Autodesk Fusion 360 part; units mm, degrees
(part 2 of 6)
  line L465 (-177.5, -38.5) -> (-158.5, -57.5) construction
  arc A308 (-137.675, -57.5) -> (-134.5, -54.325) centre (-137.675, -54.325) ccw
  line L466 (-153.5, -54.325) -> (-153.5, -41.675)
  line L467 (-134.5, -41.675) -> (-134.5, -54.325)
  line L468 (-134.5, -38.5) -> (-153.5, -57.5) construction
  arc A309 (-150.325, -38.5) -> (-153.5, -41.675) centre (-150.325, -41.675) ccw
  arc A310 (-134.5, -41.675) -> (-137.675, -38.5) centre (-137.675, -41.675) ccw
  line L469 (-137.675, -57.5) -> (-150.325, -57.5)
  line L470 (-150.325, -38.5) -> (-137.675, -38.5)
  arc A311 (-153.5, -54.325) -> (-150.325, -57.5) centre (-150.325, -54.325) ccw
  line L471 (-153.5, -38.5) -> (-134.5, -57.5) construction
  arc A312 (-113.675, -57.5) -> (-110.5, -54.325) centre (-113.675, -54.325) ccw
  line L472 (-129.5, -54.325) -> (-129.5, -41.675)
  line L473 (-110.5, -41.675) -> (-110.5, -54.325)
  line L474 (-110.5, -38.5) -> (-129.5, -57.5) construction
  arc A313 (-126.325, -38.5) -> (-129.5, -41.675) centre (-126.325, -41.675) ccw
  arc A314 (-110.5, -41.675) -> (-113.675, -38.5) centre (-113.675, -41.675) ccw
  line L475 (-113.675, -57.5) -> (-126.325, -57.5)
  line L476 (-126.325, -38.5) -> (-113.675, -38.5)
  arc A315 (-129.5, -54.325) -> (-126.325, -57.5) centre (-126.325, -54.325) ccw
  line L477 (-129.5, -38.5) -> (-110.5, -57.5) construction
  arc A316 (-89.675, -57.5) -> (-86.5, -54.325) centre (-89.675, -54.325) ccw
  line L478 (-105.5, -54.325) -> (-105.5, -41.675)
  line L479 (-86.5, -41.675) -> (-86.5, -54.325)
  line L480 (-86.5, -38.5) -> (-105.5, -57.5) construction
  arc A317 (-102.325, -38.5) -> (-105.5, -41.675) centre (-102.325, -41.675) ccw
  arc A318 (-86.5, -41.675) -> (-89.675, -38.5) centre (-89.675, -41.675) ccw
  line L481 (-89.675, -57.5) -> (-102.325, -57.5)
  line L482 (-102.325, -38.5) -> (-89.675, -38.5)
  arc A319 (-105.5, -54.325) -> (-102.325, -57.5) centre (-102.325, -54.325) ccw
  line L483 (-105.5, -38.5) -> (-86.5, -57.5) construction
  arc A320 (-65.675, -57.5) -> (-62.5, -54.325) centre (-65.675, -54.325) ccw
  line L484 (-81.5, -54.325) -> (-81.5, -41.675)
  line L485 (-62.5, -41.675) -> (-62.5, -54.325)
  line L486 (-62.5, -38.5) -> (-81.5, -57.5) construction
  arc A321 (-78.325, -38.5) -> (-81.5, -41.675) centre (-78.325, -41.675) ccw
  arc A322 (-62.5, -41.675) -> (-65.675, -38.5) centre (-65.675, -41.675) ccw
  line L487 (-65.675, -57.5) -> (-78.325, -57.5)
  line L488 (-78.325, -38.5) -> (-65.675, -38.5)
  arc A323 (-81.5, -54.325) -> (-78.325, -57.5) centre (-78.325, -54.325) ccw
  line L489 (-81.5, -38.5) -> (-62.5, -57.5) construction
  arc A324 (-41.675, -57.5) -> (-38.5, -54.325) centre (-41.675, -54.325) ccw
  line L490 (-57.5, -54.325) -> (-57.5, -41.675)
  line L491 (-38.5, -41.675) -> (-38.5, -54.325)
  line L492 (-38.5, -38.5) -> (-57.5, -57.5) construction
  arc A325 (-54.325, -38.5) -> (-57.5, -41.675) centre (-54.325, -41.675) ccw
  arc A326 (-38.5, -41.675) -> (-41.675, -38.5) centre (-41.675, -41.675) ccw
  line L493 (-41.675, -57.5) -> (-54.325, -57.5)
  line L494 (-54.325, -38.5) -> (-41.675, -38.5)
  arc A327 (-57.5, -54.325) -> (-54.325, -57.5) centre (-54.325, -54.325) ccw
  line L495 (-57.5, -38.5) -> (-38.5, -57.5) construction
  arc A328 (-17.675, -57.5) -> (-14.5, -54.325) centre (-17.675, -54.325) ccw
  line L496 (-33.5, -54.325) -> (-33.5, -41.675)
  line L497 (-14.5, -41.675) -> (-14.5, -54.325)
  line L498 (-14.5, -38.5) -> (-33.5, -57.5) construction
  arc A329 (-30.325, -38.5) -> (-33.5, -41.675) centre (-30.325, -41.675) ccw
  arc A330 (-14.5, -41.675) -> (-17.675, -38.5) centre (-17.675, -41.675) ccw
  line L499 (-17.675, -57.5) -> (-30.325, -57.5)
  line L500 (-30.325, -38.5) -> (-17.675, -38.5)
  arc A331 (-33.5, -54.325) -> (-30.325, -57.5) centre (-30.325, -54.325) ccw
  line L501 (-33.5, -38.5) -> (-14.5, -57.5) construction
  arc A332 (6.325, -57.5) -> (9.5, -54.325) centre (6.325, -54.325) ccw
  line L502 (-9.5, -54.325) -> (-9.5, -41.675)
  line L503 (9.5, -41.675) -> (9.5, -54.325)
  line L504 (9.5, -38.5) -> (-9.5, -57.5) construction
  arc A333 (-6.325, -38.5) -> (-9.5, -41.675) centre (-6.325, -41.675) ccw
  arc A334 (9.5, -41.675) -> (6.325, -38.5) centre (6.325, -41.675) ccw
  line L505 (6.325, -57.5) -> (-6.325, -57.5)
  line L506 (-6.325, -38.5) -> (6.325, -38.5)
  arc A335 (-9.5, -54.325) -> (-6.325, -57.5) centre (-6.325, -54.325) ccw
  line L507 (-9.5, -38.5) -> (9.5, -57.5) construction
  arc A336 (30.325, -57.5) -> (33.5, -54.325) centre (30.325, -54.325) ccw
  line L508 (14.5, -54.325) -> (14.5, -41.675)
  line L509 (33.5, -41.675) -> (33.5, -54.325)
  line L510 (33.5, -38.5) -> (14.5, -57.5) construction
  arc A337 (17.675, -38.5) -> (14.5, -41.675) centre (17.675, -41.675) ccw
  arc A338 (33.5, -41.675) -> (30.325, -38.5) centre (30.325, -41.675) ccw
  line L511 (30.325, -57.5) -> (17.675, -57.5)
  line L512 (17.675, -38.5) -> (30.325, -38.5)
  arc A339 (14.5, -54.325) -> (17.675, -57.5) centre (17.675, -54.325) ccw
  line L513 (14.5, -38.5) -> (33.5, -57.5) construction
  arc A340 (54.325, -57.5) -> (57.5, -54.325) centre (54.325, -54.325) ccw
  line L514 (38.5, -54.325) -> (38.5, -41.675)
  line L515 (57.5, -41.675) -> (57.5, -54.325)
  line L516 (57.5, -38.5) -> (38.5, -57.5) construction
  arc A341 (41.675, -38.5) -> (38.5, -41.675) centre (41.675, -41.675) ccw
  arc A342 (57.5, -41.675) -> (54.325, -38.5) centre (54.325, -41.675) ccw
  line L517 (54.325, -57.5) -> (41.675, -57.5)
  line L518 (41.675, -38.5) -> (54.325, -38.5)
  arc A343 (38.5, -54.325) -> (41.675, -57.5) centre (41.675, -54.325) ccw
  line L519 (38.5, -38.5) -> (57.5, -57.5) construction
  arc A344 (78.325, -57.5) -> (81.5, -54.325) centre (78.325, -54.325) ccw
  line L520 (62.5, -54.325) -> (62.5, -41.675)
  line L521 (81.5, -41.675) -> (81.5, -54.325)
  line L522 (81.5, -38.5) -> (62.5, -57.5) construction
  arc A345 (65.675, -38.5) -> (62.5, -41.675) centre (65.675, -41.675) ccw
  arc A346 (81.5, -41.675) -> (78.325, -38.5) centre (78.325, -41.675) ccw
  line L523 (78.325, -57.5) -> (65.675, -57.5)
  line L524 (65.675, -38.5) -> (78.325, -38.5)
  arc A347 (62.5, -54.325) -> (65.675, -57.5) centre (65.675, -54.325) ccw
  line L525 (62.5, -38.5) -> (81.5, -57.5) construction
  arc A348 (102.325, -57.5) -> (105.5, -54.325) centre (102.325, -54.325) ccw
  line L526 (86.5, -54.325) -> (86.5, -41.675)
  line L527 (105.5, -41.675) -> (105.5, -54.325)
  line L528 (105.5, -38.5) -> (86.5, -57.5) construction
  arc A349 (89.675, -38.5) -> (86.5, -41.675) centre (89.675, -41.675) ccw
  arc A350 (105.5, -41.675) -> (102.325, -38.5) centre (102.325, -41.675) ccw
  line L529 (102.325, -57.5) -> (89.675, -57.5)
  line L530 (89.675, -38.5) -> (102.325, -38.5)
  arc A351 (86.5, -54.325) -> (89.675, -57.5) centre (89.675, -54.325) ccw
  line L531 (86.5, -38.5) -> (105.5, -57.5) construction
  arc A352 (126.325, -57.5) -> (129.5, -54.325) centre (126.325, -54.325) ccw
  line L532 (110.5, -54.325) -> (110.5, -41.675)
  line L533 (129.5, -41.675) -> (129.5, -54.325)
  line L534 (129.5, -38.5) -> (110.5, -57.5) construction
  arc A353 (113.675, -38.5) -> (110.5, -41.675) centre (113.675, -41.675) ccw
  arc A354 (129.5, -41.675) -> (126.325, -38.5) centre (126.325, -41.675) ccw
  line L535 (126.325, -57.5) -> (113.675, -57.5)
  line L536 (113.675, -38.5) -> (126.325, -38.5)
  arc A355 (110.5, -54.325) -> (113.675, -57.5) centre (113.675, -54.325) ccw
  line L537 (110.5, -38.5) -> (129.5, -57.5) construction
  arc A356 (150.325, -57.5) -> (153.5, -54.325) centre (150.325, -54.325) ccw
  line L538 (134.5, -54.325) -> (134.5, -41.675)
  line L539 (153.5, -41.675) -> (153.5, -54.325)
  line L540 (153.5, -38.5) -> (134.5, -57.5) construction
  arc A357 (137.675, -38.5) -> (134.5, -41.675) centre (137.675, -41.675) ccw
  arc A358 (153.5, -41.675) -> (150.325, -38.5) centre (150.325, -41.675) ccw
  line L541 (150.325, -57.5) -> (137.675, -57.5)
  line L542 (137.675, -38.5) -> (150.325, -38.5)
  arc A359 (134.5, -54.325) -> (137.675, -57.5) centre (137.675, -54.325) ccw
  line L543 (134.5, -38.5) -> (153.5, -57.5) construction
  arc A360 (174.325, -57.5) -> (177.5, -54.325) centre (174.325, -54.325) ccw
  line L544 (158.5, -54.325) -> (158.5, -41.675)
  line L545 (177.5, -41.675) -> (177.5, -54.325)
  line L546 (177.5, -38.5) -> (158.5, -57.5) construction
  arc A361 (161.675, -38.5) -> (158.5, -41.675) centre (161.675, -41.675) ccw
  arc A362 (177.5, -41.675) -> (174.325, -38.5) centre (174.325, -41.675) ccw
  line L547 (174.325, -57.5) -> (161.675, -57.5)
  line L548 (161.675, -38.5) -> (174.325, -38.5)
  arc A363 (158.5, -54.325) -> (161.675, -57.5) centre (161.675, -54.325) ccw
  line L549 (158.5, -38.5) -> (177.5, -57.5) construction
  arc A364 (-161.675, -33.5) -> (-158.5, -30.325) centre (-161.675, -30.325) ccw
  line L550 (-177.5, -30.325) -> (-177.5, -17.675)
  line L551 (-158.5, -17.675) -> (-158.5, -30.325)
  line L552 (-158.5, -14.5) -> (-177.5, -33.5) construction
  arc A365 (-174.325, -14.5) -> (-177.5, -17.675) centre (-174.325, -17.675) ccw
  arc A366 (-158.5, -17.675) -> (-161.675, -14.5) centre (-161.675, -17.675) ccw
  line L553 (-161.675, -33.5) -> (-174.325, -33.5)
  line L554 (-174.325, -14.5) -> (-161.675, -14.5)
  arc A367 (-177.5, -30.325) -> (-174.325, -33.5) centre (-174.325, -30.325) ccw
  line L555 (-177.5, -14.5) -> (-158.5, -33.5) construction
  arc A368 (-137.675, -33.5) -> (-134.5, -30.325) centre (-137.675, -30.325) ccw
  line L556 (-153.5, -30.325) -> (-153.5, -17.675)
  line L557 (-134.5, -17.675) -> (-134.5, -30.325)
  line L558 (-134.5, -14.5) -> (-153.5, -33.5) construction
  arc A369 (-150.325, -14.5) -> (-153.5, -17.675) centre (-150.325, -17.675) ccw
  arc A370 (-134.5, -17.675) -> (-137.675, -14.5) centre (-137.675, -17.675) ccw
  line L559 (-137.675, -33.5) -> (-150.325, -33.5)
  line L560 (-150.325, -14.5) -> (-137.675, -14.5)
  arc A371 (-153.5, -30.325) -> (-150.325, -33.5) centre (-150.325, -30.325) ccw
  line L561 (-153.5, -14.5) -> (-134.5, -33.5) construction
  arc A372 (-113.675, -33.5) -> (-110.5, -30.325) centre (-113.675, -30.325) ccw
  line L562 (-129.5, -30.325) -> (-129.5, -17.675)
  line L563 (-110.5, -17.675) -> (-110.5, -30.325)
  line L564 (-110.5, -14.5) -> (-129.5, -33.5) construction
  arc A373 (-126.325, -14.5) -> (-129.5, -17.675) centre (-126.325, -17.675) ccw
  arc A374 (-110.5, -17.675) -> (-113.675, -14.5) centre (-113.675, -17.675) ccw
  line L565 (-113.675, -33.5) -> (-126.325, -33.5)
  line L566 (-126.325, -14.5) -> (-113.675, -14.5)
  arc A375 (-129.5, -30.325) -> (-126.325, -33.5) centre (-126.325, -30.325) ccw
  line L567 (-129.5, -14.5) -> (-110.5, -33.5) construction
  arc A376 (-89.675, -33.5) -> (-86.5, -30.325) centre (-89.675, -30.325) ccw
  line L568 (-105.5, -30.325) -> (-105.5, -17.675)
  line L569 (-86.5, -17.675) -> (-86.5, -30.325)
  line L570 (-86.5, -14.5) -> (-105.5, -33.5) construction
  arc A377 (-102.325, -14.5) -> (-105.5, -17.675) centre (-102.325, -17.675) ccw
  arc A378 (-86.5, -17.675) -> (-89.675, -14.5) centre (-89.675, -17.675) ccw
  line L571 (-89.675, -33.5) -> (-102.325, -33.5)
  line L572 (-102.325, -14.5) -> (-89.675, -14.5)
  arc A379 (-105.5, -30.325) -> (-102.325, -33.5) centre (-102.325, -30.325) ccw
  line L573 (-105.5, -14.5) -> (-86.5, -33.5) construction
  arc A380 (-65.675, -33.5) -> (-62.5, -30.325) centre (-65.675, -30.325) ccw
  line L574 (-81.5, -30.325) -> (-81.5, -17.675)
  line L575 (-62.5, -17.675) -> (-62.5, -30.325)
  line L576 (-62.5, -14.5) -> (-81.5, -33.5) construction
  arc A381 (-78.325, -14.5) -> (-81.5, -17.675) centre (-78.325, -17.675) ccw
  arc A382 (-62.5, -17.675) -> (-65.675, -14.5) centre (-65.675, -17.675) ccw
  line L577 (-65.675, -33.5) -> (-78.325, -33.5)
  line L578 (-78.325, -14.5) -> (-65.675, -14.5)
  arc A383 (-81.5, -30.325) -> (-78.325, -33.5) centre (-78.325, -30.325) ccw
  line L579 (-81.5, -14.5) -> (-62.5, -33.5) construction
  arc A384 (-41.675, -33.5) -> (-38.5, -30.325) centre (-41.675, -30.325) ccw
  line L580 (-57.5, -30.325) -> (-57.5, -17.675)
  line L581 (-38.5, -17.675) -> (-38.5, -30.325)
  line L582 (-38.5, -14.5) -> (-57.5, -33.5) construction
  arc A385 (-54.325, -14.5) -> (-57.5, -17.675) centre (-54.325, -17.675) ccw
  arc A386 (-38.5, -17.675) -> (-41.675, -14.5) centre (-41.675, -17.675) ccw
  line L583 (-41.675, -33.5) -> (-54.325, -33.5)
  line L584 (-54.325, -14.5) -> (-41.675, -14.5)
  arc A387 (-57.5, -30.325) -> (-54.325, -33.5) centre (-54.325, -30.325) ccw
  line L585 (-57.5, -14.5) -> (-38.5, -33.5) construction
  arc A388 (-17.675, -33.5) -> (-14.5, -30.325) centre (-17.675, -30.325) ccw
  line L586 (-33.5, -30.325) -> (-33.5, -17.675)
  line L587 (-14.5, -17.675) -> (-14.5, -30.325)
  line L588 (-14.5, -14.5) -> (-33.5, -33.5) construction
  arc A389 (-30.325, -14.5) -> (-33.5, -17.675) centre (-30.325, -17.675) ccw
  arc A390 (-14.5, -17.675) -> (-17.675, -14.5) centre (-17.675, -17.675) ccw
  line L589 (-17.675, -33.5) -> (-30.325, -33.5)
  line L590 (-30.325, -14.5) -> (-17.675, -14.5)
  arc A391 (-33.5, -30.325) -> (-30.325, -33.5) centre (-30.325, -30.325) ccw
  line L591 (-33.5, -14.5) -> (-14.5, -33.5) construction
  arc A392 (6.325, -33.5) -> (9.5, -30.325) centre (6.325, -30.325) ccw
  line L592 (-9.5, -30.325) -> (-9.5, -17.675)
  line L593 (9.5, -17.675) -> (9.5, -30.325)
  line L594 (9.5, -14.5) -> (-9.5, -33.5) construction
  arc A393 (-6.325, -14.5) -> (-9.5, -17.675) centre (-6.325, -17.675) ccw
  arc A394 (9.5, -17.675) -> (6.325, -14.5) centre (6.325, -17.675) ccw
  line L595 (6.325, -33.5) -> (-6.325, -33.5)
  line L596 (-6.325, -14.5) -> (6.325, -14.5)
  arc A395 (-9.5, -30.325) -> (-6.325, -33.5) centre (-6.325, -30.325) ccw
  line L597 (-9.5, -14.5) -> (9.5, -33.5) construction
  arc A396 (30.325, -33.5) -> (33.5, -30.325) centre (30.325, -30.325) ccw
  line L598 (14.5, -30.325) -> (14.5, -17.675)
  line L599 (33.5, -17.675) -> (33.5, -30.325)
  line L600 (33.5, -14.5) -> (14.5, -33.5) construction
  arc A397 (17.675, -14.5) -> (14.5, -17.675) centre (17.675, -17.675) ccw
  arc A398 (33.5, -17.675) -> (30.325, -14.5) centre (30.325, -17.675) ccw
  line L601 (30.325, -33.5) -> (17.675, -33.5)
  line L602 (17.675, -14.5) -> (30.325, -14.5)
  arc A399 (14.5, -30.325) -> (17.675, -33.5) centre (17.675, -30.325) ccw
  line L603 (14.5, -14.5) -> (33.5, -33.5) construction
  arc A400 (54.325, -33.5) -> (57.5, -30.325) centre (54.325, -30.325) ccw
  line L604 (38.5, -30.325) -> (38.5, -17.675)
  line L605 (57.5, -17.675) -> (57.5, -30.325)
  line L606 (57.5, -14.5) -> (38.5, -33.5) construction
  arc A401 (41.675, -14.5) -> (38.5, -17.675) centre (41.675, -17.675) ccw
  arc A402 (57.5, -17.675) -> (54.325, -14.5) centre (54.325, -17.675) ccw
  line L607 (54.325, -33.5) -> (41.675, -33.5)
  line L608 (41.675, -14.5) -> (54.325, -14.5)
  arc A403 (38.5, -30.325) -> (41.675, -33.5) centre (41.675, -30.325) ccw
  line L609 (38.5, -14.5) -> (57.5, -33.5) construction
  arc A404 (78.325, -33.5) -> (81.5, -30.325) centre (78.325, -30.325) ccw
  line L610 (62.5, -30.325) -> (62.5, -17.675)
  line L611 (81.5, -17.675) -> (81.5, -30.325)
  line L612 (81.5, -14.5) -> (62.5, -33.5) construction
  arc A405 (65.675, -14.5) -> (62.5, -17.675) centre (65.675, -17.675) ccw
  arc A406 (81.5, -17.675) -> (78.325, -14.5) centre (78.325, -17.675) ccw
  line L613 (78.325, -33.5) -> (65.675, -33.5)
  line L614 (65.675, -14.5) -> (78.325, -14.5)
  arc A407 (62.5, -30.325) -> (65.675, -33.5) centre (65.675, -30.325) ccw
  line L615 (62.5, -14.5) -> (81.5, -33.5) construction
  arc A408 (102.325, -33.5) -> (105.5, -30.325) centre (102.325, -30.325) ccw
  line L616 (86.5, -30.325) -> (86.5, -17.675)
  line L617 (105.5, -17.675) -> (105.5, -30.325)
  line L618 (105.5, -14.5) -> (86.5, -33.5) construction
  arc A409 (89.675, -14.5) -> (86.5, -17.675) centre (89.675, -17.675) ccw
  arc A410 (105.5, -17.675) -> (102.325, -14.5) centre (102.325, -17.675) ccw
  line L619 (102.325, -33.5) -> (89.675, -33.5)
  line L620 (89.675, -14.5) -> (102.325, -14.5)
  arc A411 (86.5, -30.325) -> (89.675, -33.5) centre (89.675, -30.325) ccw
  line L621 (86.5, -14.5) -> (105.5, -33.5) construction
  arc A412 (126.325, -33.5) -> (129.5, -30.325) centre (126.325, -30.325) ccw
  line L622 (110.5, -30.325) -> (110.5, -17.675)
  line L623 (129.5, -17.675) -> (129.5, -30.325)
  line L624 (129.5, -14.5) -> (110.5, -33.5) construction
  arc A413 (113.675, -14.5) -> (110.5, -17.675) centre (113.675, -17.675) ccw
  arc A414 (129.5, -17.675) -> (126.325, -14.5) centre (126.325, -17.675) ccw
  line L625 (126.325, -33.5) -> (113.675, -33.5)
  line L626 (113.675, -14.5) -> (126.325, -14.5)
  arc A415 (110.5, -30.325) -> (113.675, -33.5) centre (113.675, -30.325) ccw
  line L627 (110.5, -14.5) -> (129.5, -33.5) construction
  arc A416 (150.325, -33.5) -> (153.5, -30.325) centre (150.325, -30.325) ccw
  line L628 (134.5, -30.325) -> (134.5, -17.675)
  line L629 (153.5, -17.675) -> (153.5, -30.325)
  line L630 (153.5, -14.5) -> (134.5, -33.5) construction
  arc A417 (137.675, -14.5) -> (134.5, -17.675) centre (137.675, -17.675) ccw
  arc A418 (153.5, -17.675) -> (150.325, -14.5) centre (150.325, -17.675) ccw
  line L631 (150.325, -33.5) -> (137.675, -33.5)
  line L632 (137.675, -14.5) -> (150.325, -14.5)
  arc A419 (134.5, -30.325) -> (137.675, -33.5) centre (137.675, -30.325) ccw
  line L633 (134.5, -14.5) -> (153.5, -33.5) construction
  arc A420 (174.325, -33.5) -> (177.5, -30.325) centre (174.325, -30.325) ccw
  line L634 (158.5, -30.325) -> (158.5, -17.675)
  line L635 (177.5, -17.675) -> (177.5, -30.325)
  line L636 (177.5, -14.5) -> (158.5, -33.5) construction
  arc A421 (161.675, -14.5) -> (158.5, -17.675) centre (161.675, -17.675) ccw
  arc A422 (177.5, -17.675) -> (174.325, -14.5) centre (174.325, -17.675) ccw
  line L637 (174.325, -33.5) -> (161.675, -33.5)
  line L638 (161.675, -14.5) -> (174.325, -14.5)
  arc A423 (158.5, -30.325) -> (161.675, -33.5) centre (161.675, -30.325) ccw
  line L639 (158.5, -14.5) -> (177.5, -33.5) construction
  arc A424 (-161.675, -9.5) -> (-158.5, -6.325) centre (-161.675, -6.325) ccw
  line L640 (-177.5, -6.325) -> (-177.5, 6.325)
  line L641 (-158.5, 6.325) -> (-158.5, -6.325)
  line L642 (-158.5, 9.5) -> (-177.5, -9.5) construction
  arc A425 (-174.325, 9.5) -> (-177.5, 6.325) centre (-174.325, 6.325) ccw
  arc A426 (-158.5, 6.325) -> (-161.675, 9.5) centre (-161.675, 6.325) ccw
  line L643 (-161.675, -9.5) -> (-174.325, -9.5)
  line L644 (-174.325, 9.5) -> (-161.675, 9.5)
  arc A427 (-177.5, -6.325) -> (-174.325, -9.5) centre (-174.325, -6.325) ccw
  line L645 (-177.5, 9.5) -> (-158.5, -9.5) construction
  arc A428 (-137.675, -9.5) -> (-134.5, -6.325) centre (-137.675, -6.325) ccw
  line L646 (-153.5, -6.325) -> (-153.5, 6.325)
  line L647 (-134.5, 6.325) -> (-134.5, -6.325)
  line L648 (-134.5, 9.5) -> (-153.5, -9.5) construction
  arc A429 (-150.325, 9.5) -> (-153.5, 6.325) centre (-150.325, 6.325) ccw
  arc A430 (-134.5, 6.325) -> (-137.675, 9.5) centre (-137.675, 6.325) ccw
  line L649 (-137.675, -9.5) -> (-150.325, -9.5)
  line L650 (-150.325, 9.5) -> (-137.675, 9.5)
  arc A431 (-153.5, -6.325) -> (-150.325, -9.5) centre (-150.325, -6.325) ccw
  line L651 (-153.5, 9.5) -> (-134.5, -9.5) construction
  arc A432 (-113.675, -9.5) -> (-110.5, -6.325) centre (-113.675, -6.325) ccw
  line L652 (-129.5, -6.325) -> (-129.5, 6.325)
  line L653 (-110.5, 6.325) -> (-110.5, -6.325)
  line L654 (-110.5, 9.5) -> (-129.5, -9.5) construction
  arc A433 (-126.325, 9.5) -> (-129.5, 6.325) centre (-126.325, 6.325) ccw
  arc A434 (-110.5, 6.325) -> (-113.675, 9.5) centre (-113.675, 6.325) ccw
  line L655 (-113.675, -9.5) -> (-126.325, -9.5)
  line L656 (-126.325, 9.5) -> (-113.675, 9.5)
  arc A435 (-129.5, -6.325) -> (-126.325, -9.5) centre (-126.325, -6.325) ccw
  line L657 (-129.5, 9.5) -> (-110.5, -9.5) construction
  arc A436 (-89.675, -9.5) -> (-86.5, -6.325) centre (-89.675, -6.325) ccw
  line L658 (-105.5, -6.325) -> (-105.5, 6.325)
  line L659 (-86.5, 6.325) -> (-86.5, -6.325)
  line L660 (-86.5, 9.5) -> (-105.5, -9.5) construction
  arc A437 (-102.325, 9.5) -> (-105.5, 6.325) centre (-102.325, 6.325) ccw
  arc A438 (-86.5, 6.325) -> (-89.675, 9.5) centre (-89.675, 6.325) ccw
  line L661 (-89.675, -9.5) -> (-102.325, -9.5)
  line L662 (-102.325, 9.5) -> (-89.675, 9.5)
  arc A439 (-105.5, -6.325) -> (-102.325, -9.5) centre (-102.325, -6.325) ccw
  line L663 (-105.5, 9.5) -> (-86.5, -9.5) construction
  arc A440 (-65.675, -9.5) -> (-62.5, -6.325) centre (-65.675, -6.325) ccw
  line L664 (-81.5, -6.325) -> (-81.5, 6.325)
  line L665 (-62.5, 6.325) -> (-62.5, -6.325)
  line L666 (-62.5, 9.5) -> (-81.5, -9.5) construction
  arc A441 (-78.325, 9.5) -> (-81.5, 6.325) centre (-78.325, 6.325) ccw
  arc A442 (-62.5, 6.325) -> (-65.675, 9.5) centre (-65.675, 6.325) ccw
  line L667 (-65.675, -9.5) -> (-78.325, -9.5)
  line L668 (-78.325, 9.5) -> (-65.675, 9.5)
  arc A443 (-81.5, -6.325) -> (-78.325, -9.5) centre (-78.325, -6.325) ccw
  line L669 (-81.5, 9.5) -> (-62.5, -9.5) construction
  arc A444 (-41.675, -9.5) -> (-38.5, -6.325) centre (-41.675, -6.325) ccw
  line L670 (-57.5, -6.325) -> (-57.5, 6.325)
  line L671 (-38.5, 6.325) -> (-38.5, -6.325)
  line L672 (-38.5, 9.5) -> (-57.5, -9.5) construction
  arc A445 (-54.325, 9.5) -> (-57.5, 6.325) centre (-54.325, 6.325) ccw
  arc A446 (-38.5, 6.325) -> (-41.675, 9.5) centre (-41.675, 6.325) ccw
  line L673 (-41.675, -9.5) -> (-54.325, -9.5)
  line L674 (-54.325, 9.5) -> (-41.675, 9.5)
  arc A447 (-57.5, -6.325) -> (-54.325, -9.5) centre (-54.325, -6.325) ccw
  line L675 (-57.5, 9.5) -> (-38.5, -9.5) construction
  arc A448 (-17.675, -9.5) -> (-14.5, -6.325) centre (-17.675, -6.325) ccw
  line L676 (-33.5, -6.325) -> (-33.5, 6.325)
  line L677 (-14.5, 6.325) -> (-14.5, -6.325)
  line L678 (-14.5, 9.5) -> (-33.5, -9.5) construction
  arc A449 (-30.325, 9.5) -> (-33.5, 6.325) centre (-30.325, 6.325) ccw
  arc A450 (-14.5, 6.325) -> (-17.675, 9.5) centre (-17.675, 6.325) ccw
  line L679 (-17.675, -9.5) -> (-30.325, -9.5)
  line L680 (-30.325, 9.5) -> (-17.675, 9.5)
  arc A451 (-33.5, -6.325) -> (-30.325, -9.5) centre (-30.325, -6.325) ccw
  line L681 (-33.5, 9.5) -> (-14.5, -9.5) construction
  arc A452 (30.325, -9.5) -> (33.5, -6.325) centre (30.325, -6.325) ccw
  line L682 (14.5, -6.325) -> (14.5, 6.325)
  line L683 (33.5, 6.325) -> (33.5, -6.325)
  line L684 (33.5, 9.5) -> (14.5, -9.5) construction
  arc A453 (17.675, 9.5) -> (14.5, 6.325) centre (17.675, 6.325) ccw
  arc A454 (33.5, 6.325) -> (30.325, 9.5) centre (30.325, 6.325) ccw
  line L685 (30.325, -9.5) -> (17.675, -9.5)
  line L686 (17.675, 9.5) -> (30.325, 9.5)
  arc A455 (14.5, -6.325) -> (17.675, -9.5) centre (17.675, -6.325) ccw
  line L687 (14.5, 9.5) -> (33.5, -9.5) construction
  arc A456 (54.325, -9.5) -> (57.5, -6.325) centre (54.325, -6.325) ccw
  line L688 (38.5, -6.325) -> (38.5, 6.325)
  line L689 (57.5, 6.325) -> (57.5, -6.325)
  line L690 (57.5, 9.5) -> (38.5, -9.5) construction
  arc A457 (41.675, 9.5) -> (38.5, 6.325) centre (41.675, 6.325) ccw
  arc A458 (57.5, 6.325) -> (54.325, 9.5) centre (54.325, 6.325) ccw
  line L691 (54.325, -9.5) -> (41.675, -9.5)
  line L692 (41.675, 9.5) -> (54.325, 9.5)
  arc A459 (38.5, -6.325) -> (41.675, -9.5) centre (41.675, -6.325) ccw
  line L693 (38.5, 9.5) -> (57.5, -9.5) construction
  arc A460 (78.325, -9.5) -> (81.5, -6.325) centre (78.325, -6.325) ccw
  line L694 (62.5, -6.325) -> (62.5, 6.325)
  line L695 (81.5, 6.325) -> (81.5, -6.325)
  line L696 (81.5, 9.5) -> (62.5, -9.5) construction
  arc A461 (65.675, 9.5) -> (62.5, 6.325) centre (65.675, 6.325) ccw
  arc A462 (81.5, 6.325) -> (78.325, 9.5) centre (78.325, 6.325) ccw
  line L697 (78.325, -9.5) -> (65.675, -9.5)
  line L698 (65.675, 9.5) -> (78.325, 9.5)
  arc A463 (62.5, -6.325) -> (65.675, -9.5) centre (65.675, -6.325) ccw
  line L699 (62.5, 9.5) -> (81.5, -9.5) construction
  arc A464 (102.325, -9.5) -> (105.5, -6.325) centre (102.325, -6.325) ccw
  line L700 (86.5, -6.325) -> (86.5, 6.325)
  line L701 (105.5, 6.325) -> (105.5, -6.325)
  line L702 (105.5, 9.5) -> (86.5, -9.5) construction
  arc A465 (89.675, 9.5) -> (86.5, 6.325) centre (89.675, 6.325) ccw
  arc A466 (105.5, 6.325) -> (102.325, 9.5) centre (102.325, 6.325) ccw
  line L703 (102.325, -9.5) -> (89.675, -9.5)
  line L704 (89.675, 9.5) -> (102.325, 9.5)
  arc A467 (86.5, -6.325) -> (89.675, -9.5) centre (89.675, -6.325) ccw
  line L705 (86.5, 9.5) -> (105.5, -9.5) construction
  arc A468 (126.325, -9.5) -> (129.5, -6.325) centre (126.325, -6.325) ccw
  line L706 (110.5, -6.325) -> (110.5, 6.325)
  line L707 (129.5, 6.325) -> (129.5, -6.325)
  line L708 (129.5, 9.5) -> (110.5, -9.5) construction
  arc A469 (113.675, 9.5) -> (110.5, 6.325) centre (113.675, 6.325) ccw
  arc A470 (129.5, 6.325) -> (126.325, 9.5) centre (126.325, 6.325) ccw
  line L709 (126.325, -9.5) -> (113.675, -9.5)
  line L710 (113.675, 9.5) -> (126.325, 9.5)
  arc A471 (110.5, -6.325) -> (113.675, -9.5) centre (113.675, -6.325) ccw
  line L711 (110.5, 9.5) -> (129.5, -9.5) construction
  arc A472 (150.325, -9.5) -> (153.5, -6.325) centre (150.325, -6.325) ccw
  line L712 (134.5, -6.325) -> (134.5, 6.325)
  line L713 (153.5, 6.325) -> (153.5, -6.325)
  line L714 (153.5, 9.5) -> (134.5, -9.5) construction
  arc A473 (137.675, 9.5) -> (134.5, 6.325) centre (137.675, 6.325) ccw
  arc A474 (153.5, 6.325) -> (150.325, 9.5) centre (150.325, 6.325) ccw
  line L715 (150.325, -9.5) -> (137.675, -9.5)
  line L716 (137.675, 9.5) -> (150.325, 9.5)
  arc A475 (134.5, -6.325) -> (137.675, -9.5) centre (137.675, -6.325) ccw
  line L717 (134.5, 9.5) -> (153.5, -9.5) construction
  arc A476 (174.325, -9.5) -> (177.5, -6.325) centre (174.325, -6.325) ccw
  line L718 (158.5, -6.325) -> (158.5, 6.325)
  line L719 (177.5, 6.325) -> (177.5, -6.325)
  line L720 (177.5, 9.5) -> (158.5, -9.5) construction
  arc A477 (161.675, 9.5) -> (158.5, 6.325) centre (161.675, 6.325) ccw
  arc A478 (177.5, 6.325) -> (174.325, 9.5) centre (174.325, 6.325) ccw
  line L721 (174.325, -9.5) -> (161.675, -9.5)
  line L722 (161.675, 9.5) -> (174.325, 9.5)
  arc A479 (158.5, -6.325) -> (161.675, -9.5) centre (161.675, -6.325) ccw
  line L723 (158.5, 9.5) -> (177.5, -9.5) construction
  arc A480 (-161.675, 14.5) -> (-158.5, 17.675) centre (-161.675, 17.675) ccw
  line L724 (-177.5, 17.675) -> (-177.5, 30.325)
  line L725 (-158.5, 30.325) -> (-158.5, 17.675)
  line L726 (-158.5, 33.5) -> (-177.5, 14.5) construction
  arc A481 (-174.325, 33.5) -> (-177.5, 30.325) centre (-174.325, 30.325) ccw
  arc A482 (-158.5, 30.325) -> (-161.675, 33.5) centre (-161.675, 30.325) ccw
  line L727 (-161.675, 14.5) -> (-174.325, 14.5)
  line L728 (-174.325, 33.5) -> (-161.675, 33.5)
  arc A483 (-177.5, 17.675) -> (-174.325, 14.5) centre (-174.325, 17.675) ccw
  line L729 (-177.5, 33.5) -> (-158.5, 14.5) construction
  arc A484 (-137.675, 14.5) -> (-134.5, 17.675) centre (-137.675, 17.675) ccw
  line L730 (-153.5, 17.675) -> (-153.5, 30.325)
  line L731 (-134.5, 30.325) -> (-134.5, 17.675)
  line L732 (-134.5, 33.5) -> (-153.5, 14.5) construction
  arc A485 (-150.325, 33.5) -> (-153.5, 30.325) centre (-150.325, 30.325) ccw
  arc A486 (-134.5, 30.325) -> (-137.675, 33.5) centre (-137.675, 30.325) ccw
  line L733 (-137.675, 14.5) -> (-150.325, 14.5)
  line L734 (-150.325, 33.5) -> (-137.675, 33.5)
  arc A487 (-153.5, 17.675) -> (-150.325, 14.5) centre (-150.325, 17.675) ccw
  line L735 (-153.5, 33.5) -> (-134.5, 14.5) construction
  arc A488 (-113.675, 14.5) -> (-110.5, 17.675) centre (-113.675, 17.675) ccw
  line L736 (-129.5, 17.675) -> (-129.5, 30.325)
  line L737 (-110.5, 30.325) -> (-110.5, 17.675)
  line L738 (-110.5, 33.5) -> (-129.5, 14.5) construction
  arc A489 (-126.325, 33.5) -> (-129.5, 30.325) centre (-126.325, 30.325) ccw
  arc A490 (-110.5, 30.325) -> (-113.675, 33.5) centre (-113.675, 30.325) ccw
  line L739 (-113.675, 14.5) -> (-126.325, 14.5)
  line L740 (-126.325, 33.5) -> (-113.675, 33.5)
  arc A491 (-129.5, 17.675) -> (-126.325, 14.5) centre (-126.325, 17.675) ccw
  line L741 (-129.5, 33.5) -> (-110.5, 14.5) construction
  arc A492 (-89.675, 14.5) -> (-86.5, 17.675) centre (-89.675, 17.675) ccw
  line L742 (-105.5, 17.675) -> (-105.5, 30.325)
  line L743 (-86.5, 30.325) -> (-86.5, 17.675)
  line L744 (-86.5, 33.5) -> (-105.5, 14.5) construction
  arc A493 (-102.325, 33.5) -> (-105.5, 30.325) centre (-102.325, 30.325) ccw
  arc A494 (-86.5, 30.325) -> (-89.675, 33.5) centre (-89.675, 30.325) ccw
  line L745 (-89.675, 14.5) -> (-102.325, 14.5)
  line L746 (-102.325, 33.5) -> (-89.675, 33.5)
  arc A495 (-105.5, 17.675) -> (-102.325, 14.5) centre (-102.325, 17.675) ccw
  line L747 (-105.5, 33.5) -> (-86.5, 14.5) construction
  arc A496 (-65.675, 14.5) -> (-62.5, 17.675) centre (-65.675, 17.675) ccw
  line L748 (-81.5, 17.675) -> (-81.5, 30.325)
  line L749 (-62.5, 30.325) -> (-62.5, 17.675)
  line L750 (-62.5, 33.5) -> (-81.5, 14.5) construction
  arc A497 (-78.325, 33.5) -> (-81.5, 30.325) centre (-78.325, 30.325) ccw
  arc A498 (-62.5, 30.325) -> (-65.675, 33.5) centre (-65.675, 30.325) ccw
  line L751 (-65.675, 14.5) -> (-78.325, 14.5)
  line L752 (-78.325, 33.5) -> (-65.675, 33.5)
  arc A499 (-81.5, 17.675) -> (-78.325, 14.5) centre (-78.325, 17.675) ccw
  line L753 (-81.5, 33.5) -> (-62.5, 14.5) construction
  arc A500 (-41.675, 14.5) -> (-38.5, 17.675) centre (-41.675, 17.675) ccw
  line L754 (-57.5, 17.675) -> (-57.5, 30.325)
  line L755 (-38.5, 30.325) -> (-38.5, 17.675)
  line L756 (-38.5, 33.5) -> (-57.5, 14.5) construction
  arc A501 (-54.325, 33.5) -> (-57.5, 30.325) centre (-54.325, 30.325) ccw
  arc A502 (-38.5, 30.325) -> (-41.675, 33.5) centre (-41.675, 30.325) ccw
  line L757 (-41.675, 14.5) -> (-54.325, 14.5)
  line L758 (-54.325, 33.5) -> (-41.675, 33.5)
  arc A503 (-57.5, 17.675) -> (-54.325, 14.5) centre (-54.325, 17.675) ccw
  line L759 (-57.5, 33.5) -> (-38.5, 14.5) construction
  arc A504 (-17.675, 14.5) -> (-14.5, 17.675) centre (-17.675, 17.675) ccw
  line L760 (-33.5, 17.675) -> (-33.5, 30.325)
  line L761 (-14.5, 30.325) -> (-14.5, 17.675)
  line L762 (-14.5, 33.5) -> (-33.5, 14.5) construction
  arc A505 (-30.325, 33.5) -> (-33.5, 30.325) centre (-30.325, 30.325) ccw
  arc A506 (-14.5, 30.325) -> (-17.675, 33.5) centre (-17.675, 30.325) ccw
  line L763 (-17.675, 14.5) -> (-30.325, 14.5)
  line L764 (-30.325, 33.5) -> (-17.675, 33.5)
  arc A507 (-33.5, 17.675) -> (-30.325, 14.5) centre (-30.325, 17.675) ccw
  line L765 (-33.5, 33.5) -> (-14.5, 14.5) construction
  arc A508 (6.325, 14.5) -> (9.5, 17.675) centre (6.325, 17.675) ccw
  line L766 (-9.5, 17.675) -> (-9.5, 30.325)
  line L767 (9.5, 30.325) -> (9.5, 17.675)
  line L768 (9.5, 33.5) -> (-9.5, 14.5) construction
  arc A509 (-6.325, 33.5) -> (-9.5, 30.325) centre (-6.325, 30.325) ccw
  arc A510 (9.5, 30.325) -> (6.325, 33.5) centre (6.325, 30.325) ccw
  line L769 (6.325, 14.5) -> (-6.325, 14.5)
  line L770 (-6.325, 33.5) -> (6.325, 33.5)
  arc A511 (-9.5, 17.675) -> (-6.325, 14.5) centre (-6.325, 17.675) ccw
  line L771 (-9.5, 33.5) -> (9.5, 14.5) construction
  arc A512 (30.325, 14.5) -> (33.5, 17.675) centre (30.325, 17.675) ccw
  line L772 (14.5, 17.675) -> (14.5, 30.325)
  line L773 (33.5, 30.325) -> (33.5, 17.675)
  line L774 (33.5, 33.5) -> (14.5, 14.5) construction
  arc A513 (17.675, 33.5) -> (14.5, 30.325) centre (17.675, 30.325) ccw
  arc A514 (33.5, 30.325) -> (30.325, 33.5) centre (30.325, 30.325) ccw
  line L775 (30.325, 14.5) -> (17.675, 14.5)
  line L776 (17.675, 33.5) -> (30.325, 33.5)
  arc A515 (14.5, 17.675) -> (17.675, 14.5) centre (17.675, 17.675) ccw
  line L777 (14.5, 33.5) -> (33.5, 14.5) construction
  arc A516 (54.325, 14.5) -> (57.5, 17.675) centre (54.325, 17.675) ccw
  line L778 (38.5, 17.675) -> (38.5, 30.325)
  line L779 (57.5, 30.325) -> (57.5, 17.675)
  line L780 (57.5, 33.5) -> (38.5, 14.5) construction
  arc A517 (41.675, 33.5) -> (38.5, 30.325) centre (41.675, 30.325) ccw
  arc A518 (57.5, 30.325) -> (54.325, 33.5) centre (54.325, 30.325) ccw
  line L781 (54.325, 14.5) -> (41.675, 14.5)
  line L782 (41.675, 33.5) -> (54.325, 33.5)
  arc A519 (38.5, 17.675) -> (41.675, 14.5) centre (41.675, 17.675) ccw
  line L783 (38.5, 33.5) -> (57.5, 14.5) construction
  arc A520 (78.325, 14.5) -> (81.5, 17.675) centre (78.325, 17.675) ccw
  line L784 (62.5, 17.675) -> (62.5, 30.325)
  line L785 (81.5, 30.325) -> (81.5, 17.675)
  line L786 (81.5, 33.5) -> (62.5, 14.5) construction
  arc A521 (65.675, 33.5) -> (62.5, 30.325) centre (65.675, 30.325) ccw
  arc A522 (81.5, 30.325) -> (78.325, 33.5) centre (78.325, 30.325) ccw
  line L787 (78.325, 14.5) -> (65.675, 14.5)
  line L788 (65.675, 33.5) -> (78.325, 33.5)
  arc A523 (62.5, 17.675) -> (65.675, 14.5) centre (65.675, 17.675) ccw
  line L789 (62.5, 33.5) -> (81.5, 14.5) construction
  arc A524 (102.325, 14.5) -> (105.5, 17.675) centre (102.325, 17.675) ccw
  line L790 (86.5, 17.675) -> (86.5, 30.325)
  line L791 (105.5, 30.325) -> (105.5, 17.675)
  line L792 (105.5, 33.5) -> (86.5, 14.5) construction
  arc A525 (89.675, 33.5) -> (86.5, 30.325) centre (89.675, 30.325) ccw
  arc A526 (105.5, 30.325) -> (102.325, 33.5) centre (102.325, 30.325) ccw
  line L793 (102.325, 14.5) -> (89.675, 14.5)
  line L794 (89.675, 33.5) -> (102.325, 33.5)
  arc A527 (86.5, 17.675) -> (89.675, 14.5) centre (89.675, 17.675) ccw
  line L795 (86.5, 33.5) -> (105.5, 14.5) construction
  arc A528 (126.325, 14.5) -> (129.5, 17.675) centre (126.325, 17.675) ccw
  line L796 (110.5, 17.675) -> (110.5, 30.325)
  line L797 (129.5, 30.325) -> (129.5, 17.675)
  line L798 (129.5, 33.5) -> (110.5, 14.5) construction
  arc A529 (113.675, 33.5) -> (110.5, 30.325) centre (113.675, 30.325) ccw
  arc A530 (129.5, 30.325) -> (126.325, 33.5) centre (126.325, 30.325) ccw
  line L799 (126.325, 14.5) -> (113.675, 14.5)
  line L800 (113.675, 33.5) -> (126.325, 33.5)
  arc A531 (110.5, 17.675) -> (113.675, 14.5) centre (113.675, 17.675) ccw
  line L801 (110.5, 33.5) -> (129.5, 14.5) construction
  arc A532 (150.325, 14.5) -> (153.5, 17.675) centre (150.325, 17.675) ccw
  line L802 (134.5, 17.675) -> (134.5, 30.325)
  line L803 (153.5, 30.325) -> (153.5, 17.675)
  line L804 (153.5, 33.5) -> (134.5, 14.5) construction
  arc A533 (137.675, 33.5) -> (134.5, 30.325) centre (137.675, 30.325) ccw
  arc A534 (153.5, 30.325) -> (150.325, 33.5) centre (150.325, 30.325) ccw
  line L805 (150.325, 14.5) -> (137.675, 14.5)
  line L806 (137.675, 33.5) -> (150.325, 33.5)
  arc A535 (134.5, 17.675) -> (137.675, 14.5) centre (137.675, 17.675) ccw
  line L807 (134.5, 33.5) -> (153.5, 14.5) construction
  arc A536 (174.325, 14.5) -> (177.5, 17.675) centre (174.325, 17.675) ccw
  line L808 (158.5, 17.675) -> (158.5, 30.325)
  line L809 (177.5, 30.325) -> (177.5, 17.675)
  line L810 (177.5, 33.5) -> (158.5, 14.5) construction
  arc A537 (161.675, 33.5) -> (158.5, 30.325) centre (161.675, 30.325) ccw
  arc A538 (177.5, 30.325) -> (174.325, 33.5) centre (174.325, 30.325) ccw
  line L811 (174.325, 14.5) -> (161.675, 14.5)
  line L812 (161.675, 33.5) -> (174.325, 33.5)
  arc A539 (158.5, 17.675) -> (161.675, 14.5) centre (161.675, 17.675) ccw
  line L813 (158.5, 33.5) -> (177.5, 14.5) construction
  arc A540 (-161.675, 38.5) -> (-158.5, 41.675) centre (-161.675, 41.675) ccw
  line L814 (-177.5, 41.675) -> (-177.5, 54.325)
  line L815 (-158.5, 54.325) -> (-158.5, 41.675)
  line L816 (-158.5, 57.5) -> (-177.5, 38.5) construction
  arc A541 (-174.325, 57.5) -> (-177.5, 54.325) centre (-174.325, 54.325) ccw
  arc A542 (-158.5, 54.325) -> (-161.675, 57.5) centre (-161.675, 54.325) ccw
  line L817 (-161.675, 38.5) -> (-174.325, 38.5)
  line L818 (-174.325, 57.5) -> (-161.675, 57.5)
  arc A543 (-177.5, 41.675) -> (-174.325, 38.5) centre (-174.325, 41.675) ccw
  line L819 (-177.5, 57.5) -> (-158.5, 38.5) construction
  arc A544 (-137.675, 38.5) -> (-134.5, 41.675) centre (-137.675, 41.675) ccw
  line L820 (-153.5, 41.675) -> (-153.5, 54.325)
  line L821 (-134.5, 54.325) -> (-134.5, 41.675)
  line L822 (-134.5, 57.5) -> (-153.5, 38.5) construction
  arc A545 (-150.325, 57.5) -> (-153.5, 54.325) centre (-150.325, 54.325) ccw
  arc A546 (-134.5, 54.325) -> (-137.675, 57.5) centre (-137.675, 54.325) ccw
  line L823 (-137.675, 38.5) -> (-150.325, 38.5)
  line L824 (-150.325, 57.5) -> (-137.675, 57.5)
  arc A547 (-153.5, 41.675) -> (-150.325, 38.5) centre (-150.325, 41.675) ccw
  line L825 (-153.5, 57.5) -> (-134.5, 38.5) construction
  arc A548 (-113.675, 38.5) -> (-110.5, 41.675) centre (-113.675, 41.675) ccw
  line L826 (-129.5, 41.675) -> (-129.5, 54.325)
  line L827 (-110.5, 54.325) -> (-110.5, 41.675)
  line L828 (-110.5, 57.5) -> (-129.5, 38.5) construction
  arc A549 (-126.325, 57.5) -> (-129.5, 54.325) centre (-126.325, 54.325) ccw
  arc A550 (-110.5, 54.325) -> (-113.675, 57.5) centre (-113.675, 54.325) ccw
  line L829 (-113.675, 38.5) -> (-126.325, 38.5)
  line L830 (-126.325, 57.5) -> (-113.675, 57.5)
  arc A551 (-129.5, 41.675) -> (-126.325, 38.5) centre (-126.325, 41.675) ccw
  line L831 (-129.5, 57.5) -> (-110.5, 38.5) construction
  arc A552 (-89.675, 38.5) -> (-86.5, 41.675) centre (-89.675, 41.675) ccw
  line L832 (-105.5, 41.675) -> (-105.5, 54.325)
  line L833 (-86.5, 54.325) -> (-86.5, 41.675)
  line L834 (-86.5, 57.5) -> (-105.5, 38.5) construction
  arc A553 (-102.325, 57.5) -> (-105.5, 54.325) centre (-102.325, 54.325) ccw
  arc A554 (-86.5, 54.325) -> (-89.675, 57.5) centre (-89.675, 54.325) ccw
  line L835 (-89.675, 38.5) -> (-102.325, 38.5)
  line L836 (-102.325, 57.5) -> (-89.675, 57.5)
  arc A555 (-105.5, 41.675) -> (-102.325, 38.5) centre (-102.325, 41.675) ccw
  line L837 (-105.5, 57.5) -> (-86.5, 38.5) construction
  arc A556 (-65.675, 38.5) -> (-62.5, 41.675) centre (-65.675, 41.675) ccw
  line L838 (-81.5, 41.675) -> (-81.5, 54.325)
  line L839 (-62.5, 54.325) -> (-62.5, 41.675)
  line L840 (-62.5, 57.5) -> (-81.5, 38.5) construction
  arc A557 (-78.325, 57.5) -> (-81.5, 54.325) centre (-78.325, 54.325) ccw
  arc A558 (-62.5, 54.325) -> (-65.675, 57.5) centre (-65.675, 54.325) ccw
  line L841 (-65.675, 38.5) -> (-78.325, 38.5)
  line L842 (-78.325, 57.5) -> (-65.675, 57.5)
  arc A559 (-81.5, 41.675) -> (-78.325, 38.5) centre (-78.325, 41.675) ccw
  line L843 (-81.5, 57.5) -> (-62.5, 38.5) construction
  arc A560 (-41.675, 38.5) -> (-38.5, 41.675) centre (-41.675, 41.675) ccw
  line L844 (-57.5, 41.675) -> (-57.5, 54.325)
  line L845 (-38.5, 54.325) -> (-38.5, 41.675)
  line L846 (-38.5, 57.5) -> (-57.5, 38.5) construction
  arc A561 (-54.325, 57.5) -> (-57.5, 54.325) centre (-54.325, 54.325) ccw
  arc A562 (-38.5, 54.325) -> (-41.675, 57.5) centre (-41.675, 54.325) ccw
  line L847 (-41.675, 38.5) -> (-54.325, 38.5)
  line L848 (-54.325, 57.5) -> (-41.675, 57.5)
  arc A563 (-57.5, 41.675) -> (-54.325, 38.5) centre (-54.325, 41.675) ccw
  line L849 (-57.5, 57.5) -> (-38.5, 38.5) construction
  arc A564 (-17.675, 38.5) -> (-14.5, 41.675) centre (-17.675, 41.675) ccw
  line L850 (-33.5, 41.675) -> (-33.5, 54.325)
  line L851 (-14.5, 54.325) -> (-14.5, 41.675)
  line L852 (-14.5, 57.5) -> (-33.5, 38.5) construction
  arc A565 (-30.325, 57.5) -> (-33.5, 54.325) centre (-30.325, 54.325) ccw
  arc A566 (-14.5, 54.325) -> (-17.675, 57.5) centre (-17.675, 54.325) ccw
  line L853 (-17.675, 38.5) -> (-30.325, 38.5)
  line L854 (-30.325, 57.5) -> (-17.675, 57.5)
  arc A567 (-33.5, 41.675) -> (-30.325, 38.5) centre (-30.325, 41.675) ccw
  line L855 (-33.5, 57.5) -> (-14.5, 38.5) construction
  arc A568 (6.325, 38.5) -> (9.5, 41.675) centre (6.325, 41.675) ccw
  line L856 (-9.5, 41.675) -> (-9.5, 54.325)
  line L857 (9.5, 54.325) -> (9.5, 41.675)
  line L858 (9.5, 57.5) -> (-9.5, 38.5) construction
  arc A569 (-6.325, 57.5) -> (-9.5, 54.325) centre (-6.325, 54.325) ccw
  arc A570 (9.5, 54.325) -> (6.325, 57.5) centre (6.325, 54.325) ccw
  line L859 (6.325, 38.5) -> (-6.325, 38.5)
  line L860 (-6.325, 57.5) -> (6.325, 57.5)
  arc A571 (-9.5, 41.675) -> (-6.325, 38.5) centre (-6.325, 41.675) ccw
  line L861 (-9.5, 57.5) -> (9.5, 38.5) construction
  arc A572 (30.325, 38.5) -> (33.5, 41.675) centre (30.325, 41.675) ccw
  line L862 (14.5, 41.675) -> (14.5, 54.325)
  line L863 (33.5, 54.325) -> (33.5, 41.675)
  line L864 (33.5, 57.5) -> (14.5, 38.5) construction
  arc A573 (17.675, 57.5) -> (14.5, 54.325) centre (17.675, 54.325) ccw
  arc A574 (33.5, 54.325) -> (30.325, 57.5) centre (30.325, 54.325) ccw
  line L865 (30.325, 38.5) -> (17.675, 38.5)
  line L866 (17.675, 57.5) -> (30.325, 57.5)
  arc A575 (14.5, 41.675) -> (17.675, 38.5) centre (17.675, 41.675) ccw
  line L867 (14.5, 57.5) -> (33.5, 38.5) construction
  arc A576 (54.325, 38.5) -> (57.5, 41.675) centre (54.325, 41.675) ccw
  line L868 (38.5, 41.675) -> (38.5, 54.325)
  line L869 (57.5, 54.325) -> (57.5, 41.675)
  line L870 (57.5, 57.5) -> (38.5, 38.5) construction
  arc A577 (41.675, 57.5) -> (38.5, 54.325) centre (41.675, 54.325) ccw
  arc A578 (57.5, 54.325) -> (54.325, 57.5) centre (54.325, 54.325) ccw
  line L871 (54.325, 38.5) -> (41.675, 38.5)
  line L872 (41.675, 57.5) -> (54.325, 57.5)
  arc A579 (38.5, 41.675) -> (41.675, 38.5) centre (41.675, 41.675) ccw
  line L873 (38.5, 57.5) -> (57.5, 38.5) construction
  arc A580 (78.325, 38.5) -> (81.5, 41.675) centre (78.325, 41.675) ccw
  line L874 (62.5, 41.675) -> (62.5, 54.325)
  line L875 (81.5, 54.325) -> (81.5, 41.675)
  line L876 (81.5, 57.5) -> (62.5, 38.5) construction
  arc A581 (65.675, 57.5) -> (62.5, 54.325) centre (65.675, 54.325) ccw
  arc A582 (81.5, 54.325) -> (78.325, 57.5) centre (78.325, 54.325) ccw
  line L877 (78.325, 38.5) -> (65.675, 38.5)
  line L878 (65.675, 57.5) -> (78.325, 57.5)
  arc A583 (62.5, 41.675) -> (65.675, 38.5) centre (65.675, 41.675) ccw
  line L879 (62.5, 57.5) -> (81.5, 38.5) construction
  arc A584 (102.325, 38.5) -> (105.5, 41.675) centre (102.325, 41.675) ccw
  line L880 (86.5, 41.675) -> (86.5, 54.325)
  line L881 (105.5, 54.325) -> (105.5, 41.675)
  line L882 (105.5, 57.5) -> (86.5, 38.5) construction
  arc A585 (89.675, 57.5) -> (86.5, 54.325) centre (89.675, 54.325) ccw
  arc A586 (105.5, 54.325) -> (102.325, 57.5) centre (102.325, 54.325) ccw
  line L883 (102.325, 38.5) -> (89.675, 38.5)
  line L884 (89.675, 57.5) -> (102.325, 57.5)
  arc A587 (86.5, 41.675) -> (89.675, 38.5) centre (89.675, 41.675) ccw
  line L885 (86.5, 57.5) -> (105.5, 38.5) construction
  arc A588 (126.325, 38.5) -> (129.5, 41.675) centre (126.325, 41.675) ccw
  line L886 (110.5, 41.675) -> (110.5, 54.325)
  line L887 (129.5, 54.325) -> (129.5, 41.675)
  line L888 (129.5, 57.5) -> (110.5, 38.5) construction
  arc A589 (113.675, 57.5) -> (110.5, 54.325) centre (113.675, 54.325) ccw
  arc A590 (129.5, 54.325) -> (126.325, 57.5) centre (126.325, 54.325) ccw
  line L889 (126.325, 38.5) -> (113.675, 38.5)
  line L890 (113.675, 57.5) -> (126.325, 57.5)
  arc A591 (110.5, 41.675) -> (113.675, 38.5) centre (113.675, 41.675) ccw
  line L891 (110.5, 57.5) -> (129.5, 38.5) construction
  arc A592 (150.325, 38.5) -> (153.5, 41.675) centre (150.325, 41.675) ccw
  line L892 (134.5, 41.675) -> (134.5, 54.325)
  line L893 (153.5, 54.325) -> (153.5, 41.675)
  line L894 (153.5, 57.5) -> (134.5, 38.5) construction
  arc A593 (137.675, 57.5) -> (134.5, 54.325) centre (137.675, 54.325) ccw
  arc A594 (153.5, 54.325) -> (150.325, 57.5) centre (150.325, 54.325) ccw
  line L895 (150.325, 38.5) -> (137.675, 38.5)
  line L896 (137.675, 57.5) -> (150.325, 57.5)
  arc A595 (134.5, 41.675) -> (137.675, 38.5) centre (137.675, 41.675) ccw
  line L897 (134.5, 57.5) -> (153.5, 38.5) construction
  arc A596 (174.325, 38.5) -> (177.5, 41.675) centre (174.325, 41.675) ccw
  line L898 (158.5, 41.675) -> (158.5, 54.325)
  line L899 (177.5, 54.325) -> (177.5, 41.675)
  line L900 (177.5, 57.5) -> (158.5, 38.5) construction
  arc A597 (161.675, 57.5) -> (158.5, 54.325) centre (161.675, 54.325) ccw
  arc A598 (177.5, 54.325) -> (174.325, 57.5) centre (174.325, 54.325) ccw
  line L901 (174.325, 38.5) -> (161.675, 38.5)
  line L902 (161.675, 57.5) -> (174.325, 57.5)
  arc A599 (158.5, 41.675) -> (161.675, 38.5) centre (161.675, 41.675) ccw
  line L903 (158.5, 57.5) -> (177.5, 38.5) construction
  arc A600 (-161.675, 62.5) -> (-158.5, 65.675) centre (-161.675, 65.675) ccw
  line L904 (-177.5, 65.675) -> (-177.5, 78.325)
  line L905 (-158.5, 78.325) -> (-158.5, 65.675)
  line L906 (-158.5, 81.5) -> (-177.5, 62.5) construction
  arc A601 (-174.325, 81.5) -> (-177.5, 78.325) centre (-174.325, 78.325) ccw
  arc A602 (-158.5, 78.325) -> (-161.675, 81.5) centre (-161.675, 78.325) ccw
  line L907 (-161.675, 62.5) -> (-174.325, 62.5)
  line L908 (-174.325, 81.5) -> (-161.675, 81.5)
  arc A603 (-177.5, 65.675) -> (-174.325, 62.5) centre (-174.325, 65.675) ccw
  line L909 (-177.5, 81.5) -> (-158.5, 62.5) construction
  arc A604 (-137.675, 62.5) -> (-134.5, 65.675) centre (-137.675, 65.675) ccw
  line L910 (-153.5, 65.675) -> (-153.5, 78.325)
  line L911 (-134.5, 78.325) -> (-134.5, 65.675)
  line L912 (-134.5, 81.5) -> (-153.5, 62.5) construction
  arc A605 (-150.325, 81.5) -> (-153.5, 78.325) centre (-150.325, 78.325) ccw
  arc A606 (-134.5, 78.325) -> (-137.675, 81.5) centre (-137.675, 78.325) ccw
  line L913 (-137.675, 62.5) -> (-150.325, 62.5)
  line L914 (-150.325, 81.5) -> (-137.675, 81.5)
  arc A607 (-153.5, 65.675) -> (-150.325, 62.5) centre (-150.325, 65.675) ccw
  line L915 (-153.5, 81.5) -> (-134.5, 62.5) construction
  arc A608 (-113.675, 62.5) -> (-110.5, 65.675) centre (-113.675, 65.675) ccw
  line L916 (-129.5, 65.675) -> (-129.5, 78.325)
  line L917 (-110.5, 78.325) -> (-110.5, 65.675)
  line L918 (-110.5, 81.5) -> (-129.5, 62.5) construction
  arc A609 (-126.325, 81.5) -> (-129.5, 78.325) centre (-126.325, 78.325) ccw
  arc A610 (-110.5, 78.325) -> (-113.675, 81.5) centre (-113.675, 78.325) ccw
  line L919 (-113.675, 62.5) -> (-126.325, 62.5)
  line L920 (-126.325, 81.5) -> (-113.675, 81.5)
  arc A611 (-129.5, 65.675) -> (-126.325, 62.5) centre (-126.325, 65.675) ccw
  line L921 (-129.5, 81.5) -> (-110.5, 62.5) construction
  arc A612 (-89.675, 62.5) -> (-86.5, 65.675) centre (-89.675, 65.675) ccw
  line L922 (-105.5, 65.675) -> (-105.5, 78.325)
  line L923 (-86.5, 78.325) -> (-86.5, 65.675)
  line L924 (-86.5, 81.5) -> (-105.5, 62.5) construction
  arc A613 (-102.325, 81.5) -> (-105.5, 78.325) centre (-102.325, 78.325) ccw
  arc A614 (-86.5, 78.325) -> (-89.675, 81.5) centre (-89.675, 78.325) ccw
  line L925 (-89.675, 62.5) -> (-102.325, 62.5)
  line L926 (-102.325, 81.5) -> (-89.675, 81.5)
  arc A615 (-105.5, 65.675) -> (-102.325, 62.5) centre (-102.325, 65.675) ccw
  line L927 (-105.5, 81.5) -> (-86.5, 62.5) construction
  arc A616 (-65.675, 62.5) -> (-62.5, 65.675) centre (-65.675, 65.675) ccw
  line L928 (-81.5, 65.675) -> (-81.5, 78.325)
  line L929 (-62.5, 78.325) -> (-62.5, 65.675)
  line L930 (-62.5, 81.5) -> (-81.5, 62.5) construction
  arc A617 (-78.325, 81.5) -> (-81.5, 78.325) centre (-78.325, 78.325) ccw
  arc A618 (-62.5, 78.325) -> (-65.675, 81.5) centre (-65.675, 78.325) ccw
  line L931 (-65.675, 62.5) -> (-78.325, 62.5)
  line L932 (-78.325, 81.5) -> (-65.675, 81.5)
  arc A619 (-81.5, 65.675) -> (-78.325, 62.5) centre (-78.325, 65.675) ccw
  line L933 (-81.5, 81.5) -> (-62.5, 62.5) construction
  arc A620 (-41.675, 62.5) -> (-38.5, 65.675) centre (-41.675, 65.675) ccw
  line L934 (-57.5, 65.675) -> (-57.5, 78.325)
  line L935 (-38.5, 78.325) -> (-38.5, 65.675)
  line L936 (-38.5, 81.5) -> (-57.5, 62.5) construction
  arc A621 (-54.325, 81.5) -> (-57.5, 78.325) centre (-54.325, 78.325) ccw
  arc A622 (-38.5, 78.325) -> (-41.675, 81.5) centre (-41.675, 78.325) ccw
  line L937 (-41.675, 62.5) -> (-54.325, 62.5)
  line L938 (-54.325, 81.5) -> (-41.675, 81.5)
  arc A623 (-57.5, 65.675) -> (-54.325, 62.5) centre (-54.325, 65.675) ccw
  line L939 (-57.5, 81.5) -> (-38.5, 62.5) construction
  arc A624 (-17.675, 62.5) -> (-14.5, 65.675) centre (-17.675, 65.675) ccw
  line L940 (-33.5, 65.675) -> (-33.5, 78.325)
  line L941 (-14.5, 78.325) -> (-14.5, 65.675)
  line L942 (-14.5, 81.5) -> (-33.5, 62.5) construction
  arc A625 (-30.325, 81.5) -> (-33.5, 78.325) centre (-30.325, 78.325) ccw
  arc A626 (-14.5, 78.325) -> (-17.675, 81.5) centre (-17.675, 78.325) ccw
  line L943 (-17.675, 62.5) -> (-30.325, 62.5)
  line L944 (-30.325, 81.5) -> (-17.675, 81.5)
  arc A627 (-33.5, 65.675) -> (-30.325, 62.5) centre (-30.325, 65.675) ccw
  line L945 (-33.5, 81.5) -> (-14.5, 62.5) construction
  arc A628 (6.325, 62.5) -> (9.5, 65.675) centre (6.325, 65.675) ccw
  line L946 (-9.5, 65.675) -> (-9.5, 78.325)
  line L947 (9.5, 78.325) -> (9.5, 65.675)
  line L948 (9.5, 81.5) -> (-9.5, 62.5) construction
  arc A629 (-6.325, 81.5) -> (-9.5, 78.325) centre (-6.325, 78.325) ccw
  arc A630 (9.5, 78.325) -> (6.325, 81.5) centre (6.325, 78.325) ccw
  line L949 (6.325, 62.5) -> (-6.325, 62.5)
  line L950 (-6.325, 81.5) -> (6.325, 81.5)
  arc A631 (-9.5, 65.675) -> (-6.325, 62.5) centre (-6.325, 65.675) ccw
  line L951 (-9.5, 81.5) -> (9.5, 62.5) construction
  arc A632 (30.325, 62.5) -> (33.5, 65.675) centre (30.325, 65.675) ccw
  line L952 (14.5, 65.675) -> (14.5, 78.325)
  line L953 (33.5, 78.325) -> (33.5, 65.675)
  line L954 (33.5, 81.5) -> (14.5, 62.5) construction
  arc A633 (17.675, 81.5) -> (14.5, 78.325) centre (17.675, 78.325) ccw
  arc A634 (33.5, 78.325) -> (30.325, 81.5) centre (30.325, 78.325) ccw
  line L955 (30.325, 62.5) -> (17.675, 62.5)
  line L956 (17.675, 81.5) -> (30.325, 81.5)
  arc A635 (14.5, 65.675) -> (17.675, 62.5) centre (17.675, 65.675) ccw
  line L957 (14.5, 81.5) -> (33.5, 62.5) construction
  arc A636 (54.325, 62.5) -> (57.5, 65.675) centre (54.325, 65.675) ccw
  line L958 (38.5, 65.675) -> (38.5, 78.325)
  line L959 (57.5, 78.325) -> (57.5, 65.675)
  line L960 (57.5, 81.5) -> (38.5, 62.5) construction